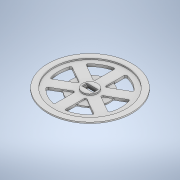
# Autodesk Inventor part: FS-03-SLBV1
Saved by Autodesk Inventor 2022 (Build 260153000, 153)
## iProperties
Created: 2022-01-12
Part Number: FS-03-SLBV1
Material: Generic
Document SubType Name: Modeling
Designer: Frank
Density: 1 g/cm^3
Appearance: Default
Author: Frank
Autodesk Inventor part; units mm, degrees
ref_plane "YZ Plane" through (0, 0, 0) normal (1, 0, 0) x (0, 1, 0)
ref_plane "XZ Plane" through (0, 0, 0) normal (0, 1, 0) x (-1, 0, 0)
ref_plane "XY Plane" through (0, 0, 0) normal (0, 0, 1) x (1, 0, 0)
sketch "Sketch1" plane through (0, 0, 0) normal (1, 0, 0) x (0, 1, 0)
  line L0 (0, 0) -> (-3, 0)
  line L1 (0, 28.5) -> (0, 33)
  line L2 (0, 33) -> (-1, 33)
  line L3 (-1, 33) -> (-1, 29.5)
  line L4 (-1, 29.5) -> (-3, 29.5)
  line L5 (-3, 29.5) -> (-3, 0)
  line L6 (0, 28.5) -> (-1, 28.5)
  line L7 (-1, 28.5) -> (-1, 5)
  line L8 (-2, 2.5) -> (-3, 2.5)
  line L9 (-1, 5) -> (-2, 5)
  line L10 (-2, 5) -> (-2, 0)
  line L11 (0, 33) -> (0, 0) construction
  line L12 (-1, 5) -> (0, 5)
  line L13 (-1, 6) -> (0, 6)
  line L14 (0, 5) -> (0, 6)
  line L15 (0, 6) -> (0, 0)
  line L16 (0, 0) -> (-3, 0)
  point P0 (-1, 2.5)
  point P1 (0, 5)
  dimension "d0" = 66
  dimension "d2" = 3
  dimension "d3" = 1
  dimension "d6" = 1
  dimension "d20" = 5
  dimension "d21" = 10
  dimension "d22" = 1
  dimension "d23" = 1
  dimension "d31" = 59
  dimension "d32" = 1
  constraints: 34 end point, 9 perpendicular, 5 point on line, 3 collinear, 3 vertical, 2 horizontal, 1 midpoint
  measures "d0" diameter of L2 L0
  measures "d2" distance between parallel lines of L1 L5
  measures "d3" distance of L1.end L2.end
  measures "d6" distance between parallel lines of L1 L7
  measures "d20" diameter of L8 L0
  measures "d21" diameter of L9 L0
  measures "d22" distance between parallel lines of L5 L10
  measures "d23" distance between parallel lines of L12 L13
  measures "d31" diameter of L4 L0
  measures "d32" distance from line of L1.start L4
revolve "Revolution1" add sketch "Sketch1" angle 360 about axis through (0, 0, 0) along (0, -1, 0)
sketch "Sketch2" plane through (0, -1, 0) normal (0, 1, 0) x (1, 0, 0)
  arc A0 (-24.6817, 14.25) -> (-24.6817, -14.25) centre (0, 0) ccw
  line L0 (-1.7321, -1) -> (-24.6817, -14.25)
  line L1 (-1.7321, 1) -> (-24.6817, 14.25)
  arc A1 (-1.7321, 1) -> (-1.7321, -1) centre (0, 0) ccw
  line L2 (-28.5, 0) -> (0, 0) construction
  line L3 (0, 0) -> (-24.6817, -14.25) construction
  line L4 (0, 0) -> (-24.6817, 14.25) construction
  line L5 (-21.8856, -8.0169) -> (-9.5, -0.866)
  arc A2 (-5.873, -1.228) -> (-5.873, 1.228) centre (0, 0) ccw
  line L6 (-9.5, 0.866) -> (-21.8856, 8.0169)
  arc A3 (-23.3382, 7.4551) -> (-23.3382, -7.4551) centre (0, 0) ccw
  arc A4 (-9.5, -0.866) -> (-9.5, 0.866) centre (-10, 0) ccw
  arc A5 (-21.8856, 8.0169) -> (-23.3382, 7.4551) centre (-22.3856, 7.1508) ccw
  arc A6 (-23.3382, -7.4551) -> (-21.8856, -8.0169) centre (-22.3856, -7.1508) ccw
  arc A7 (-18.1254, -16.4839) -> (-5.2128, -23.939) centre (0, 0) ccw
  arc A8 (-5.2128, -23.939) -> (-4, -22.9619) centre (-5, -22.9619) ccw
  line L7 (-4, -22.9619) -> (-4, -8.6603)
  arc A9 (-4, -8.6603) -> (-5.5, -7.7942) centre (-5, -8.6603) ccw
  line L8 (-5.5, -7.7942) -> (-17.8856, -14.9451)
  arc A10 (-17.8856, -14.9451) -> (-18.1254, -16.4839) centre (-17.3856, -15.8111) ccw
  arc A11 (5.2128, -23.939) -> (18.1254, -16.4839) centre (0, 0) ccw
  arc A12 (18.1254, -16.4839) -> (17.8856, -14.9451) centre (17.3856, -15.8111) ccw
  line L9 (17.8856, -14.9451) -> (5.5, -7.7942)
  arc A13 (5.5, -7.7942) -> (4, -8.6603) centre (5, -8.6603) ccw
  line L10 (4, -8.6603) -> (4, -22.9619)
  arc A14 (4, -22.9619) -> (5.2128, -23.939) centre (5, -22.9619) ccw
  arc A15 (23.3382, -7.4551) -> (23.3382, 7.4551) centre (0, 0) ccw
  arc A16 (23.3382, 7.4551) -> (21.8856, 8.0169) centre (22.3856, 7.1508) ccw
  line L11 (21.8856, 8.0169) -> (9.5, 0.866)
  arc A17 (9.5, 0.866) -> (9.5, -0.866) centre (10, 0) ccw
  line L12 (9.5, -0.866) -> (21.8856, -8.0169)
  arc A18 (21.8856, -8.0169) -> (23.3382, -7.4551) centre (22.3856, -7.1508) ccw
  arc A19 (18.1254, 16.4839) -> (5.2128, 23.939) centre (0, 0) ccw
  arc A20 (5.2128, 23.939) -> (4, 22.9619) centre (5, 22.9619) ccw
  line L13 (4, 22.9619) -> (4, 8.6603)
  arc A21 (4, 8.6603) -> (5.5, 7.7942) centre (5, 8.6603) ccw
  line L14 (5.5, 7.7942) -> (17.8856, 14.9451)
  arc A22 (17.8856, 14.9451) -> (18.1254, 16.4839) centre (17.3856, 15.8111) ccw
  arc A23 (-5.2128, 23.939) -> (-18.1254, 16.4839) centre (0, 0) ccw
  arc A24 (-18.1254, 16.4839) -> (-17.8856, 14.9451) centre (-17.3856, 15.8111) ccw
  line L15 (-17.8856, 14.9451) -> (-5.5, 7.7942)
  arc A25 (-5.5, 7.7942) -> (-4, 8.6603) centre (-5, 8.6603) ccw
  line L16 (-4, 8.6603) -> (-4, 22.9619)
  arc A26 (-4, 22.9619) -> (-5.2128, 23.939) centre (-5, 22.9619) ccw
  circle A27 centre (0, 0) radius 28.5 construction
  point P0 (-22.9329, -8.6215)
  point P1 (-22.9329, 8.6215)
  point P2 (-4, -4.4721)
  point P3 (-1.873, -5.7002)
  point P4 (1.873, -5.7002)
  point P5 (4, -4.4721)
  point P6 (5.873, -1.228)
  point P7 (5.873, 1.228)
  point P8 (4, 4.4721)
  point P9 (1.873, 5.7002)
  point P10 (-1.873, 5.7002)
  point P11 (-4, 4.4721)
  dimension "d7" = 60
  dimension "d8" = 2
  dimension "d13" = 4
  dimension "d15" = 1
  dimension "d18" = 360
  constraints: 57 point on circle, 34 end point, 27 centre point, 15 point on line, 6 tangent, 3 equal radius, 2 coincident, 2 collinear, 1 horizontal, 113 other
  measures "d7" angle of L1 L0
  measures "d8" radius of A1
  measures "d13" radial gap between concentric circles of A0 A3
  measures "d15" radius of A6
extrude "Extrusion1" cut sketch "Sketch2" against normal through all contours A6 A3 A5 L6 A4 L5 | A10 L8 A9 L7 A8 A7 | A14 L10 A13 L9 A12 A11 | A18 L12 A17 L11 A16 A15 | A22 L14 A21 L13 A20 A19 | A26 L16 A25 L15 A24 A23
sketch "Sketch3" plane through (0, 0, 0) normal (0, 1, 0) x (1, 0, 0)
  line L0 (3.5, -2) -> (-3.5, -2)
  line L1 (-3.5, -2) -> (-3.5, 2)
  line L2 (-3.5, 2) -> (3.5, 2)
  line L3 (3.5, 2) -> (3.5, -2)
  line L4 (3.5, -2) -> (-3.5, 2) construction
  line L5 (-3.5, -2) -> (3.5, 2) construction
  circle A0 centre (0, 0) radius 33 projected
  circle A1 centre (0, 0) radius 28.5 projected
  circle A2 centre (0, 0) radius 6 projected
  line L6 (-5.6569, -2) -> (5.6569, -2)
  circle A3 centre (0, 0) radius 6 projected
  line L7 (-5.6569, 2) -> (5.6569, 2)
  line L8 (-4.5, -2) -> (-4.5, 2)
  line L9 (4.5, 2) -> (4.5, -2)
  line L10 (0, -2) -> (0, 2) construction
  point P0 (3.5, 2)
  point P1 (3.5, -2)
  point P2 (-3.5, -2)
  point P3 (-3.5, 2)
  dimension "d24" = 4
  dimension "d27" = 9
  dimension "d36" = 7
  constraints: 22 end point, 4 midpoint, 4 point on line, 3 parallel, 3 perpendicular, 3 point on circle, 2 collinear, 2 horizontal, 3 other
  measures "d24" distance of L0.end L1.end
  measures "d27" distance between parallel lines of L9 L8
  measures "d36" distance between parallel lines of L3 L1
extrude "Extrusion2" cut sketch "Sketch3" against normal through all contours L0 L1 L2 L3
extrude "Extrusion3" cut sketch "Sketch3" against normal blind 2 contours L3 L7 L9 L6 | L6 L8 L7 L1
chamfer "Chamfer1" distance 1 angle 45 2 edges at (-4.5, -2, 0) (4.5, -2, 0)
sketch "Sketch4" plane through (0, -3, 0) normal (0, -1, 0) x (1, 0, 0)
  line L0 (-3.5, -2) -> (3.5, -2) projected
  line L1 (3.5, -2) -> (3.5, 2) projected
  line L2 (3.5, 2) -> (-3.5, 2) projected
  line L3 (-3.5, 2) -> (-3.5, -2) projected
  arc A0 (18.1254, -16.4839) -> (17.8856, -14.9451) centre (17.3856, -15.8111) ccw projected
  line L4 (17.8856, -14.9451) -> (5.5, -7.7942) projected
  arc A1 (5.5, -7.7942) -> (4, -8.6603) centre (5, -8.6603) ccw projected
  line L5 (4, -8.6603) -> (4, -22.9619) projected
  arc A2 (4, -22.9619) -> (5.2128, -23.939) centre (5, -22.9619) ccw projected
  arc A3 (5.2128, -23.939) -> (18.1254, -16.4839) centre (0, 0) ccw projected
  arc A4 (-18.1254, 16.4839) -> (-17.8856, 14.9451) centre (-17.3856, 15.8111) ccw projected
  line L6 (-17.8856, 14.9451) -> (-5.5, 7.7942) projected
  arc A5 (-5.5, 7.7942) -> (-4, 8.6603) centre (-5, 8.6603) ccw projected
  line L7 (-4, 8.6603) -> (-4, 22.9619) projected
  arc A6 (-4, 22.9619) -> (-5.2128, 23.939) centre (-5, 22.9619) ccw projected
  arc A7 (-5.2128, 23.939) -> (-18.1254, 16.4839) centre (0, 0) ccw projected
  arc A8 (-5.2128, -23.939) -> (-4, -22.9619) centre (-5, -22.9619) ccw projected
  line L8 (-4, -22.9619) -> (-4, -8.6603) projected
  arc A9 (-4, -8.6603) -> (-5.5, -7.7942) centre (-5, -8.6603) ccw projected
  line L9 (-5.5, -7.7942) -> (-17.8856, -14.9451) projected
  arc A10 (-17.8856, -14.9451) -> (-18.1254, -16.4839) centre (-17.3856, -15.8111) ccw projected
  arc A11 (-18.1254, -16.4839) -> (-5.2128, -23.939) centre (0, 0) ccw projected
  arc A12 (23.3382, 7.4551) -> (21.8856, 8.0169) centre (22.3856, 7.1508) ccw projected
  line L10 (21.8856, 8.0169) -> (9.5, 0.866) projected
  arc A13 (9.5, 0.866) -> (9.5, -0.866) centre (10, 0) ccw projected
  line L11 (9.5, -0.866) -> (21.8856, -8.0169) projected
  arc A14 (21.8856, -8.0169) -> (23.3382, -7.4551) centre (22.3856, -7.1508) ccw projected
  arc A15 (23.3382, -7.4551) -> (23.3382, 7.4551) centre (0, 0) ccw projected
  arc A16 (5.2128, 23.939) -> (4, 22.9619) centre (5, 22.9619) ccw projected
  line L12 (4, 22.9619) -> (4, 8.6603) projected
  arc A17 (4, 8.6603) -> (5.5, 7.7942) centre (5, 8.6603) ccw projected
  line L13 (5.5, 7.7942) -> (17.8856, 14.9451) projected
  arc A18 (17.8856, 14.9451) -> (18.1254, 16.4839) centre (17.3856, 15.8111) ccw projected
  arc A19 (18.1254, 16.4839) -> (5.2128, 23.939) centre (0, 0) ccw projected
  arc A20 (-21.8856, 8.0169) -> (-23.3382, 7.4551) centre (-22.3856, 7.1508) ccw projected
  arc A21 (-23.3382, 7.4551) -> (-23.3382, -7.4551) centre (0, 0) ccw projected
  arc A22 (-23.3382, -7.4551) -> (-21.8856, -8.0169) centre (-22.3856, -7.1508) ccw projected
  line L14 (-21.8856, -8.0169) -> (-9.5, -0.866) projected
  arc A23 (-9.5, -0.866) -> (-9.5, 0.866) centre (-10, 0) ccw projected
  line L15 (-9.5, 0.866) -> (-21.8856, 8.0169) projected
  circle A24 centre (0, 0) radius 29.5 projected
  circle A25 centre (0, 0) radius 15
  dimension "d33" = 30
  constraints: 1 centre point, 1 coincident
  measures "d33" diameter of A25
extrude "Extrusion4" add sketch "Sketch4" against normal blind 1 contours A25 L5 A1 L4 | L4 A1 L5 A25 L8 A9 L9 L14 A23 L15 L6 A5 L7 L12 A17 L13 L10 A13 L11 | L11 A13 L10 A25 | A25 L9 A9 L8 | A25 L15 A23 L14 | L13 A17 L12 A25 | A25 L7 A5 L6
fillet "Fillet2" radius 1 12 edges at (4, -2.5, -14.4568) (10.52, -2.5, -10.6925) (14.52, -2.5, -3.7643) (14.52, -2.5, 3.7643) (10.52, -2.5, 10.6925) (4, -2.5, 14.4568) (-4, -2.5, 14.4568) (-14.52, -2.5, -3.7643) (-4, -2.5, -14.4568) (-10.52, -2.5, -10.6925) (-14.52, -2.5, 3.7643) (-10.52, -2.5, 10.6925)
body "Solid1"
